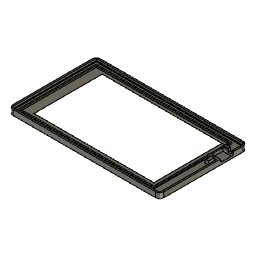
Soldered Inkplate 5 v1.2.0. Top v1.0.0. (Autodesk Fusion 360 design; units mm, degrees)
Autodesk Fusion 360 part; units mm, degrees
note: some values were not read from the file. Chosen so that the rebuilt part matches the saved one: which pieces of a blend or face edit are solid.
sketch "Sketch1" plane through (0, 0, 0) normal (0, 0, 1) x (1, 0, 0)
  line L0 (68.62, 42.115) -> (-68.62, 42.115)
  line L1 (-72.62, 38.115) -> (-72.62, -38.115)
  line L2 (-68.62, -42.115) -> (68.62, -42.115)
  line L3 (72.62, -38.115) -> (72.62, 38.115)
  line L4 (72.62, 42.115) -> (-72.62, -42.115) construction
  line L5 (-72.62, 42.115) -> (72.62, -42.115) construction
  arc A0 (-68.62, 42.115) -> (-72.62, 38.115) centre (-68.62, 38.115) ccw
  arc A1 (-72.62, -38.115) -> (-68.62, -42.115) centre (-68.62, -38.115) ccw
  arc A2 (68.62, -42.115) -> (72.62, -38.115) centre (68.62, -38.115) ccw
  arc A3 (72.62, 38.115) -> (68.62, 42.115) centre (68.62, 38.115) ccw
  line L6 (57.62, 32.765) -> (-57.62, 32.765)
  line L7 (-57.62, 32.765) -> (-57.62, -32.765)
  line L8 (-57.62, -32.765) -> (57.62, -32.765)
  line L9 (57.62, -32.765) -> (57.62, 32.765)
  line L10 (57.62, 32.765) -> (-57.62, -32.765) construction
  line L11 (-57.62, 32.765) -> (57.62, -32.765) construction
  dimension "d1" = 145.24
  dimension "d2" = 84.23
  dimension "d3" = 4
  dimension "d4" = 4
  dimension "d5" = 115.24
  dimension "d6" = 65.53
  constraint horizontal L0
  constraint perpendicular L0 L1
  constraint parallel L0 L2
  constraint parallel L1 L3
  constraint coincident L4 origin
  constraint coincident L5 origin
  constraint coincident L5.start L0
  constraint coincident L5.start L1
  constraint tangent L0 A0
  constraint tangent L1 A0
  constraint coincident L4.end L1
  constraint coincident L4.end L2
  constraint tangent L1 A1
  constraint tangent L2 A1
  constraint coincident L5.end L3
  constraint coincident L5.end L2
  constraint tangent L3 A2
  constraint tangent L2 A2
  constraint equal A1 A2
  constraint coincident L4.start L3
  constraint coincident L4.start L0
  constraint tangent L3 A3
  constraint tangent L0 A3
  constraint equal A1 A3
  constraint horizontal L6
  constraint perpendicular L6 L7
  constraint parallel L6 L8
  constraint parallel L7 L9
  constraint coincident L10 origin
  constraint coincident L11 origin
  measures "d1" distance of L4.end L5.end
  measures "d2" distance of L5.start L4.end
  measures "d3" radius of A0
  measures "d4" radius of A1
  measures "d5" distance of L6.start L6.end
  measures "d6" distance of L6.end L7.end
extrude "Extrude1" add sketch "Sketch1" along normal blind 5
sketch "Sketch2" plane through (0, 0, 5) normal (0, 0, 1) x (-1, 0, 0)
  line L0 (-57.62, -32.765) -> (-57.62, 32.765)
  line L1 (-57.62, 32.765) -> (57.62, 32.765)
  line L2 (57.62, 32.765) -> (57.62, -32.765)
  line L3 (57.62, -32.765) -> (-57.62, -32.765)
  arc A0 (-72.62, -38.115) -> (-68.62, -42.115) centre (-68.62, -38.115) ccw
  line L4 (-68.62, -42.115) -> (68.62, -42.115)
  arc A1 (68.62, -42.115) -> (72.62, -38.115) centre (68.62, -38.115) ccw
  line L5 (72.62, -38.115) -> (72.62, 38.115)
  arc A2 (72.62, 38.115) -> (68.62, 42.115) centre (68.62, 38.115) ccw
  line L6 (68.62, 42.115) -> (-68.62, 42.115)
  arc A3 (-68.62, 42.115) -> (-72.62, 38.115) centre (-68.62, 38.115) ccw
  line L7 (-72.62, 38.115) -> (-72.62, -38.115)
  line L8 (-71.12, -40.615) -> (71.12, -40.615)
  line L9 (71.12, -40.615) -> (71.12, 40.615)
  line L10 (71.12, 40.615) -> (-71.12, 40.615)
  line L11 (-71.12, 40.615) -> (-71.12, -40.615)
  line L12 (-71.12, -40.615) -> (71.12, 40.615) construction
  line L13 (71.12, -40.615) -> (-71.12, 40.615) construction
  dimension "d9" = 1.5
  dimension "d10" = 1.5
  constraint horizontal L8
  constraint perpendicular L8 L9
  constraint parallel L8 L10
  constraint parallel L9 L11
  constraint coincident L12 origin
  constraint coincident L13 origin
  measures "d9" distance of L4 L8
  measures "d10" distance of L7 L11
extrude "Extrude2" cut sketch "Sketch2" against normal blind 2.6 contours L8 L9 L10 L11
chamfer "Chamfer1" distance 2.4 angle 45 4 edges at (-57.62, 0, 0) (0, -32.765, 0) (57.62, 0, 0) (0, 32.765, 0)
sketch "Sketch3" plane through (0, 0, 2.4) normal (0, 0, 1) x (-1, 0, 0)
  line L0 (2.825, 3.2438) -> (2.825, -5) construction
  line L1 (0, 0) -> (17.5492, 0) construction
  line L2 (68.12, 37.615) -> (-62.47, 37.615)
  line L3 (-62.47, 37.615) -> (-62.47, -37.615)
  line L4 (-62.47, -37.615) -> (68.12, -37.615)
  line L5 (68.12, -37.615) -> (68.12, 37.615)
  line L6 (68.12, 37.615) -> (-62.47, -37.615) construction
  line L7 (-62.47, 37.615) -> (68.12, -37.615) construction
  line L8 (-71.12, 40.615) -> (71.12, 40.615)
  line L9 (71.12, 40.615) -> (71.12, -40.615)
  line L10 (66.12, 35.615) -> (-60.47, 35.615)
  line L11 (-60.47, 35.615) -> (-60.47, -35.615)
  line L12 (-60.47, -35.615) -> (66.12, -35.615)
  line L13 (66.12, -35.615) -> (66.12, 35.615)
  line L14 (66.12, 35.615) -> (-60.47, -35.615) construction
  line L15 (-60.47, 35.615) -> (66.12, -35.615) construction
  point P0 (2.825, 0)
  point P1 (2.825, 0)
  dimension "d21" = 2.825
  dimension "d22" = 3
  dimension "d23" = 3
  dimension "d24" = 2
  dimension "d25" = 2
  constraint vertical L0
  constraint coincident L1.start origin
  constraint perpendicular L0 L1
  constraint horizontal L2
  constraint perpendicular L2 L3
  constraint parallel L2 L4
  constraint parallel L3 L5
  constraint coincident L6 P1
  constraint coincident L7 P1
  constraint coincident L0 P1
  constraint coincident L1 P1
  constraint horizontal L10
  constraint perpendicular L10 L11
  constraint parallel L10 L12
  constraint parallel L11 L13
  constraint coincident L14 P1
  constraint coincident L15 P1
  constraint coincident P1 P0
  measures "d21" distance of L1.start L0
  measures "d22" distance of L2 L8
  measures "d23" distance of L5 L9
  measures "d24" distance of L5 L13
  measures "d25" distance of L2 L10
extrude "Extrude3" add sketch "Sketch3" along normal blind 0.74
chamfer "Chamfer2" distance 0.74 angle 45 4 edges at (-2.825, -35.615, 3.14) (60.47, 0, 3.14) (-66.12, 0, 3.14) (-2.825, 35.615, 3.14)
sketch "Sketch4" plane through (0, 0, 2.4) normal (0, 0, 1) x (-1, 0, 0)
  line L0 (-71.12, 40.615) -> (-71.12, -40.615)
  line L1 (-71.12, -40.615) -> (71.12, -40.615)
  line L2 (71.12, -40.615) -> (71.12, 40.615)
  line L3 (71.12, 40.615) -> (-71.12, 40.615)
  line L4 (68.12, -37.615) -> (-62.47, -37.615)
  line L5 (-62.47, -37.615) -> (-62.47, 37.615)
  line L6 (-62.47, 37.615) -> (68.12, 37.615)
  line L7 (68.12, 37.615) -> (68.12, -37.615)
  line L8 (-77, -29.115) -> (-76, -29.115)
  line L9 (-76, -29.115) -> (-55, -29.115) construction
  line L10 (-68.62, -42.115) -> (68.62, -42.115)
  line L11 (-78, -16.115) -> (-55, -16.115) construction
  line L12 (-67.62, -14) -> (-67.62, -35) construction
  line L13 (-71.12, -16.115) -> (-62.47, -16.115)
  line L14 (-62.47, -16.115) -> (-62.47, -14.115)
  line L15 (-62.47, -14.115) -> (-71.12, -14.115)
  line L16 (-71.12, -14.115) -> (-71.12, -16.115)
  line L17 (-67.62, -29.115) -> (-62.47, -29.115)
  line L18 (-62.47, -29.115) -> (-62.47, -31.115)
  line L19 (-62.47, -31.115) -> (-67.62, -31.115)
  line L20 (-67.62, -31.115) -> (-67.62, -29.115)
  dimension "d29" = 13
  dimension "d30" = 13
  dimension "d31" = 3.5
  dimension "d32" = 2
  dimension "d33" = 2
  constraint perpendicular L0 L8
  constraint perpendicular L0 L9
  constraint horizontal L11
  constraint perpendicular L9 L12
  constraint horizontal L13
  constraint vertical L14
  constraint horizontal L15
  constraint vertical L16
  constraint coincident L5 L14.end
  constraint coincident L11 L13.start
  constraint coincident L0 L13.start
  constraint horizontal L17
  constraint vertical L18
  constraint horizontal L19
  constraint vertical L20
  constraint coincident L5 L18.end
  constraint coincident L9 L17.start
  constraint coincident L12 L17.start
  measures "d29" distance of L9 L10
  measures "d30" distance of L9 L11
  measures "d31" distance of L0 L12
  measures "d32" distance of L13.start L15.end
  measures "d33" distance of L17.start L19.end
extrude "Extrude4" add sketch "Sketch4" along normal blind 2.6 contours L0 L5 L13 L14 L15 L16 | L5 L17 L18 L19 L20
sketch "Sketch5" plane through (72.62, 0, 0) normal (1, 0, 0) x (0, 1, 0)
  line L0 (-38.115, 0) -> (38.115, 0)
  line L1 (38.115, 0) -> (38.115, 5)
  line L2 (38.115, 5) -> (-38.115, 5)
  line L3 (-38.115, 5) -> (-38.115, 0)
  line L4 (29.115, 8) -> (29.115, -5) construction
  line L5 (29.115, 5) -> (16.115, 5)
  line L6 (16.115, 5) -> (16.115, 2)
  line L7 (16.115, 2) -> (29.115, 2)
  line L8 (29.115, 2) -> (29.115, 5)
  point P0 (42.115, 5)
  dimension "d36" = 13
  dimension "d37" = 13
  dimension "d38" = 3
  constraint perpendicular L2 L4
  constraint horizontal L5
  constraint vertical L6
  constraint horizontal L7
  constraint vertical L8
  constraint coincident L4 L5.start
  constraint coincident L2 L5.start
  measures "d36" distance of L4 P0
  measures "d37" distance of L5.start L5.end
  measures "d38" distance of L5.start L7.end
extrude "Extrude5" cut sketch "Sketch5" against normal blind 10.15 contours L2 L5 L6 L7 L8
fillet "Fillet1" radius 2 3 edges at (62.47, 22.615, 2) (67.545, 16.115, 2) (67.545, 29.115, 2)
sketch "Sketch6" plane through (0, 0, 5) normal (0, 0, 1) x (-1, 0, 0)
  line L0 (-71.12, -29.115) -> (-72.62, -29.115)
  line L1 (-72.62, -29.115) -> (-72.62, -38.115)
  arc A0 (-72.62, -38.115) -> (-68.62, -42.115) centre (-68.62, -38.115) ccw
  line L2 (-68.62, -42.115) -> (68.62, -42.115)
  arc A1 (68.62, -42.115) -> (72.62, -38.115) centre (68.62, -38.115) ccw
  line L3 (72.62, -38.115) -> (72.62, 38.115)
  arc A2 (72.62, 38.115) -> (68.62, 42.115) centre (68.62, 38.115) ccw
  line L4 (68.62, 42.115) -> (-68.62, 42.115)
  arc A3 (-68.62, 42.115) -> (-72.62, 38.115) centre (-68.62, 38.115) ccw
  line L5 (-72.62, 38.115) -> (-72.62, -16.115)
  line L6 (-72.62, -16.115) -> (-62.47, -16.115)
  line L7 (-62.47, -16.115) -> (-62.47, -14.115)
  line L8 (-62.47, -14.115) -> (-71.12, -14.115)
  line L9 (-71.12, -14.115) -> (-71.12, 40.615)
  line L10 (-71.12, 40.615) -> (71.12, 40.615)
  line L11 (71.12, 40.615) -> (71.12, -40.615)
  line L12 (71.12, -40.615) -> (-71.12, -40.615)
  line L13 (-71.12, -40.615) -> (-71.12, -29.115)
  line L14 (-71.12, -40.615) -> (71.12, -40.615)
  line L15 (71.12, -40.615) -> (71.12, 40.615)
  line L16 (71.12, 40.615) -> (-71.12, 40.615)
  line L17 (-71.12, 40.615) -> (-71.12, -40.615)
  line L18 (-70.12, -39.615) -> (70.12, -39.615)
  line L19 (70.12, -39.615) -> (70.12, 39.615)
  line L20 (70.12, 39.615) -> (-70.12, 39.615)
  line L21 (-70.12, 39.615) -> (-70.12, -39.615)
  line L22 (-71.12, -29.115) -> (-70.12, -29.115)
  line L23 (-71.12, -14.115) -> (-70.12, -14.115)
  line L24 (-70.12, -13.615) -> (-71.12, -13.615)
  dimension "d43" = 1
  dimension "d44" = 1
  dimension "d45" = 1
  dimension "d46" = 1
  dimension "d51" = 0.5
  constraint horizontal L14
  constraint vertical L15
  constraint horizontal L16
  constraint vertical L17
  constraint coincident L10.end L11.start
  constraint coincident L12.end L13.start
  constraint horizontal L18
  constraint vertical L19
  constraint horizontal L20
  constraint vertical L21
  constraint coincident L0.start L13.end
  constraint coincident L21 L22.end
  constraint perpendicular L21 L22
  constraint coincident L8.end L9.start
  constraint coincident L8 L23.end
  constraint coincident L21 L23.end
  constraint coincident L21 L24.start
  constraint coincident L17 L24.end
  constraint horizontal L24
  measures "d43" distance of L15 L19
  measures "d44" distance of L16 L20
  measures "d45" distance of L14 L18
  measures "d46" distance of L17 L21
  measures "d51" distance of L23 L24
extrude "Extrude6" add sketch "Sketch6" against normal blind 2 contours L9 L10 L11 L12 L13 L14 L15 L16 L17 L18 L19 L20 L21 L22 L24
chamfer "Chamfer3" distance 1 distance2 1 10 edges at (70.12, 34.365, 3) (0, 39.615, 3) (70.12, -13, 3) (-70.12, 0, 3) (0, -39.615, 3) (70.12, 34.365, 5) (0, 39.615, 5) (70.12, -13, 5) (0, -39.615, 5) (-70.12, 0, 5) measured on face at (-23.3733, 40.2817, 3) measured on face at (-23.3733, 40.2817, 3) measured on face at (-23.3733, 40.2817, 3) measured on face at (-23.3733, 40.2817, 3) measured on face at (-23.3733, 40.2817, 3) measured on face at (70.12, 32.615, 4.3333) measured on face at (23.3733, 39.615, 3.6667) measured on face at (70.12, -21.8717, 4.3333) measured on face at (-23.3733, -39.615, 3.6667) measured on face at (-70.12, 13.205, 3.6667)
extrude "Extrude7" cut 1 faces at (68.2367, -21.3717, 2.4) along direction (0, 0, -1) blind 0.4
sketch "Sketch7" plane through (0, 0, 2) normal (0, 0, 1) x (-1, 0, 0)
  line L0 (-71.12, -28.315) -> (-71.12, -40.615)
  line L1 (-71.12, -40.615) -> (71.12, -40.615)
  line L2 (71.12, -40.615) -> (71.12, 40.615)
  line L3 (71.12, 40.615) -> (-71.12, 40.615)
  line L4 (-71.12, 40.615) -> (-71.12, -14.115)
  line L5 (-71.12, -14.115) -> (-62.47, -14.115)
  line L6 (-62.47, -14.115) -> (-62.47, 37.615)
  line L7 (-62.47, 37.615) -> (68.12, 37.615)
  line L8 (68.12, 37.615) -> (68.12, -37.615)
  line L9 (68.12, -37.615) -> (-62.47, -37.615)
  line L10 (-62.47, -37.615) -> (-62.47, -31.115)
  line L11 (-62.47, -31.115) -> (-67.62, -31.115)
  line L12 (-67.62, -31.115) -> (-67.62, -28.315)
  line L13 (-67.62, -28.315) -> (-71.12, -28.315)
  line L14 (-65.47, -14.115) -> (-68.97, -14.115)
  line L15 (-68.97, -14.115) -> (-68.97, -8.615)
  line L16 (-68.97, -8.615) -> (-65.47, -8.615)
  line L17 (-65.47, -8.615) -> (-65.47, -14.115)
  line L18 (-72.62, 38.115) -> (-72.62, -16.115)
  dimension "d57" = 3.5
  dimension "d58" = 5.5
  dimension "d60" = 3
  constraint horizontal L14
  constraint vertical L15
  constraint horizontal L16
  constraint vertical L17
  constraint coincident L5 L14.end
  measures "d57" distance of L14.start L14.end
  measures "d58" distance of L14.start L16.end
  measures "d60" distance of L6 L17
extrude "Extrude8" add sketch "Sketch7" along normal blind 3.5 contours L5 L14 L15 L16 L17
chamfer "Chamfer5" distance 0.6 distance2 0.6 1 edges at (65.47, 11.365, 5.5) measured on face at (67.8033, 10.4483, 5.5)
equation "d5 = 114.24 mm + 1 mm"
equation "d6 = 64.53 mm + 1 mm"
